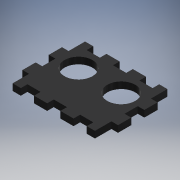
# Autodesk Inventor part: front
Saved by Autodesk Inventor 2019 (Build 230136000, 136)
## iProperties
Created: 2018-06-06
Part Number: front
Material: PBT Plastic Black
Document SubType Name: Modeling
Designer: stra92745
Density: 1.31 g/cm^3
Appearance: Smooth - White
Author: stra92745
Autodesk Inventor part; units mm, degrees
ref_plane "YZ Plane" through (0, 0, 0) normal (1, 0, 0) x (0, 1, 0)
ref_plane "XZ Plane" through (0, 0, 0) normal (0, 1, 0) x (-1, 0, 0)
ref_plane "XY Plane" through (0, 0, 0) normal (0, 0, 1) x (1, 0, 0)
sketch "Sketch1" plane through (0, 0, 0) normal (0, 1, 0) x (-1, 0, 0)
  line L0 (0, 0) -> (-58, 0)
  line L1 (-58, 0) -> (-58, -44)
  line L2 (-58, -44) -> (0, -44)
  line L3 (0, -44) -> (0, 0)
  circle A0 centre (-16, -28) radius 8.5
  circle A1 centre (-42, -28) radius 8.5
  line L4 (-16, -28) -> (-42, -28) construction
  dimension "d0" = 58
  dimension "d1" = 44
  dimension "d2" = 17
  dimension "d3" = 16
  dimension "d4" = 16
  dimension "d18" = 26
  constraints: 10 end point, 2 centre point, 2 horizontal, 2 parallel, 1 equal radius, 1 perpendicular
  measures "d0" distance of L2.end L1.end
  measures "d1" distance of L1.end L0.end
  measures "d2" diameter of A0
  measures "d3" distance from line of L2 L4.start
  measures "d4" distance from line of L3 L4.start
  measures "d18" distance of L4.start L4.end
extrude "Extrusion1" add sketch "Sketch1" along normal blind 4
sketch "Sketch2" plane through (0, 4, 0) normal (0, 1, 0) x (1, 0, 0)
  line L0 (58, 44) -> (0, 44) projected
  line L1 (0, 44) -> (0, 0) projected
  line L2 (0, 0) -> (58, 0) projected
  line L3 (58, 0) -> (58, 44) projected
  line L4 (4, 40) -> (54, 40)
  line L5 (54, 40) -> (54, 4)
  line L6 (54, 4) -> (4, 4)
  line L7 (4, 4) -> (4, 40)
  line L8 (4, 44) -> (4, 34)
  line L9 (4, 34) -> (0, 34)
  line L10 (0, 44) -> (4, 44)
  line L11 (0, 34) -> (0, 44)
  line L12 (0, 22) -> (58, 22) construction
  line L13 (4, 26) -> (0, 26)
  line L14 (0, 26) -> (0, 22)
  line L15 (4, 26) -> (4, 22)
  line L16 (29, 22) -> (29, 44) construction
  line L17 (9, 44) -> (9, 40)
  line L18 (9, 40) -> (17, 40)
  line L19 (17, 40) -> (17, 44)
  line L20 (9, 44) -> (17, 44)
  line L21 (25, 44) -> (25, 40)
  line L22 (29, 40) -> (25, 40)
  line L23 (25, 44) -> (29, 44)
  line L24 (54, 44) -> (54, 34)
  line L25 (54, 34) -> (58, 34)
  line L26 (58, 44) -> (54, 44)
  line L27 (58, 34) -> (58, 44)
  line L28 (54, 26) -> (58, 26)
  line L29 (58, 26) -> (58, 22)
  line L30 (54, 26) -> (54, 22)
  line L31 (49, 44) -> (49, 40)
  line L32 (49, 40) -> (41, 40)
  line L33 (41, 40) -> (41, 44)
  line L34 (49, 44) -> (41, 44)
  line L35 (33, 44) -> (33, 40)
  line L36 (29, 40) -> (33, 40)
  line L37 (33, 44) -> (29, 44)
  line L38 (58, 0) -> (0, 0)
  line L39 (4, 4) -> (54, 4)
  line L40 (4, 0) -> (4, 10)
  line L41 (4, 10) -> (0, 10)
  line L42 (0, 0) -> (4, 0)
  line L43 (0, 10) -> (0, 0)
  line L44 (4, 18) -> (0, 18)
  line L45 (0, 18) -> (0, 22)
  line L46 (4, 18) -> (4, 22)
  line L47 (29, 22) -> (29, 0) construction
  line L48 (9, 0) -> (9, 4)
  line L49 (9, 4) -> (17, 4)
  line L50 (17, 4) -> (17, 0)
  line L51 (9, 0) -> (17, 0)
  line L52 (25, 0) -> (25, 4)
  line L53 (29, 4) -> (25, 4)
  line L54 (25, 0) -> (29, 0)
  line L55 (58, 18) -> (58, 22)
  line L56 (54, 18) -> (54, 22)
  line L57 (54, 10) -> (58, 10)
  line L58 (58, 10) -> (58, 0)
  line L59 (58, 0) -> (54, 0)
  line L60 (29, 4) -> (33, 4)
  line L61 (33, 0) -> (33, 4)
  line L62 (33, 0) -> (29, 0)
  line L63 (54, 18) -> (58, 18)
  line L64 (54, 0) -> (54, 10)
  line L65 (49, 4) -> (41, 4)
  line L66 (41, 4) -> (41, 0)
  line L67 (49, 0) -> (49, 4)
  line L68 (49, 0) -> (41, 0)
  dimension "d8" = 4
  dimension "d11" = 8
  dimension "d12" = 8
  dimension "d13" = 4
  dimension "d16" = 4
  dimension "d17" = 8
  constraints: 130 end point, 36 symmetric about line, 21 point on line, 7 midpoint, 5 collinear, 5 perpendicular, 2 vertical, 3 other
  measures "d8" distance between parallel lines of L0 L4
  measures "d11" distance of L17.end L18.end
  measures "d12" distance between parallel lines of L21 L19
  measures "d13" distance between parallel lines of L16 L21
  measures "d16" distance between parallel lines of L12 L13
  measures "d17" distance between parallel lines of L13 L9
extrude "Extrusion2" cut sketch "Sketch2" against normal up to surface (4 mm away) contours L3 L25 L5 L24 L0 | L31 L4 L33 L0 | L3 L63 L5 L28 | L35 L4 L21 L0 | L3 L2 L64 L5 L57 | L19 L4 L17 L0 | L2 L66 L6 L67 | L8 L7 L9 L1 L0 | L2 L52 L6 L61 | L13 L7 L44 L1 | L2 L48 L6 L50 | L41 L7 L40 L2 L1
body "Solid1"
